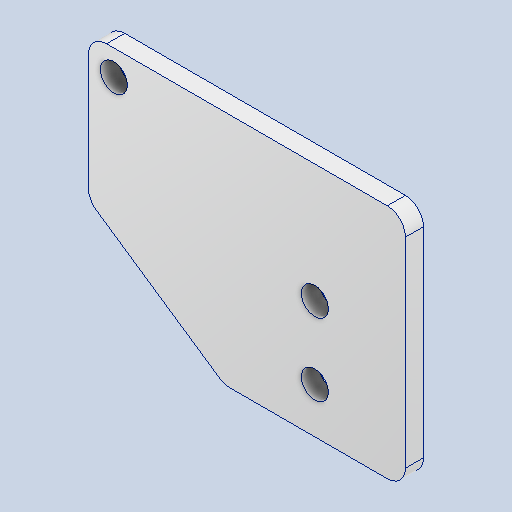
# Autodesk Inventor part: dribl-v1-Plate-12
Saved by Autodesk Inventor 2025.2 (Build 292293000, 293)
## iProperties
Created: 2025-01-15
Part Number: dribl-v1-Plate-12
Material: アルミニウム 6061
Document SubType Name: Modeling
Designer: haruy
Density: 2.7 g/cm^3
Appearance: アルミニウム - フラット
Author: haruy
Autodesk Inventor part; units mm, degrees
ref_plane "YZ Plane" through (0, 0, 0) normal (1, 0, 0) x (0, 1, 0)
ref_plane "XZ Plane" through (0, 0, 0) normal (0, 1, 0) x (-1, 0, 0)
ref_plane "XY Plane" through (0, 0, 0) normal (0, 0, 1) x (1, 0, 0)
sketch "スケッチ1" plane through (0, 0, 0) normal (0, 0, 1) x (1, 0, 0)
  line L0 (207.1172, 661.0147) -> (207.1172, -646.9853)
  line L1 (207.1172, 628.8147) -> (187.1172, 628.8147)
  line L2 (187.1172, 661.0147) -> (187.1172, -646.9853)
  line L3 (187.1172, 25.0147) -> (207.1172, 25.0147)
  line L4 (187.1172, -646.9853) -> (207.1172, -646.9853)
  line L5 (187.1172, 661.0147) -> (207.1172, 661.0147)
  line L6 (172.1172, 612.9147) -> (199.9172, 612.9147)
  line L7 (199.9172, 612.9147) -> (199.9172, 628.8147)
  line L8 (199.9172, 628.8147) -> (172.1172, 628.8147)
  line L9 (172.1172, 628.8147) -> (172.1172, 612.9147)
  circle A0 centre (174.9172, 615.7147) radius 1.5
  circle A1 centre (197.1172, 626.0147) radius 1.5
  circle A2 centre (197.1172, 634.0147) radius 1.5
  line L10 (172.1172, 79.1147) -> (199.9172, 79.1147)
  line L11 (199.9172, 79.1147) -> (199.9172, 63.2147)
  line L12 (199.9172, 63.2147) -> (172.1172, 63.2147)
  line L13 (172.1172, 63.2147) -> (172.1172, 79.1147)
  circle A3 centre (174.9172, 76.3147) radius 1.5
  circle A4 centre (197.1172, 66.0147) radius 1.5
  circle A5 centre (197.1172, 58.0147) radius 1.5
  line L14 (187.1172, 639.0147) -> (207.1172, 639.0147)
  line L15 (199.9172, 612.9147) -> (207.1172, 612.9147)
  line L16 (207.1172, 612.9147) -> (207.1172, 639.0147)
  line L17 (187.1172, 639.0147) -> (172.1172, 628.8147)
  line L18 (187.1172, 53.0147) -> (207.1172, 53.0147)
  line L19 (199.9172, 79.1147) -> (207.1172, 79.1147)
  line L20 (207.1172, 79.1147) -> (207.1172, 53.0147)
  line L21 (187.1172, 53.0147) -> (172.1172, 63.2147)
  point P0 (0, 0)
  point P1 (-212.8828, -214.6519)
  dimension "d0" = 672
  dimension "d1" = 27.8
  dimension "d2" = 15.9
  dimension "d3" = 3
  dimension "d4" = 3
  dimension "d5" = 2.8
  dimension "d6" = 2.8
  dimension "d7" = 2.8
  dimension "d8" = 2.8
  dimension "d9" = 0
  dimension "d10" = 10
  dimension "d11" = 3
  dimension "d12" = 8
  dimension "d13" = 10
  dimension "d14" = 27
  dimension "d15" = 27.8
  dimension "d16" = 15.9
  dimension "d17" = 3
  dimension "d18" = 3
  dimension "d19" = 2.8
  dimension "d20" = 2.8
  dimension "d21" = 2.8
  dimension "d22" = 2.8
  dimension "d23" = 10
  dimension "d24" = 560
  dimension "d25" = 3
  dimension "d26" = 8
  dimension "d27" = 10
  dimension "d28" = 5
  dimension "d29" = 5
  constraints: 44 end point, 10 point on line, 7 perpendicular, 6 centre point, 5 horizontal, 4 parallel
  measures "d0" distance between parallel lines of L4 L3
  measures "d1" distance of L8.end L7.end
  measures "d2" distance of L7.end L6.end
  measures "d3" diameter of A0
  measures "d4" diameter of A1
  measures "d5" distance from line of A0.centre L6
  measures "d6" distance from line of A0.centre L9
  measures "d7" distance from line of A1.centre L8
  measures "d8" distance from line of L7 A1.centre
  measures "d9" distance between parallel lines of L1 L8
  measures "d10" distance from line of A1.centre L2
  measures "d11" diameter of A2
  measures "d12" distance of A1.centre A2.centre
  measures "d13" distance from line of L2 A2.centre
  measures "d14" distance from line of A2.centre L5
  measures "d15" distance of L11.end L12.end
  measures "d16" distance of L10.end L11.end
  measures "d17" diameter of A3
  measures "d18" diameter of A4
  measures "d19" distance from line of A3.centre L10
  measures "d20" distance from line of A3.centre L13
  measures "d21" distance from line of A4.centre L12
  measures "d22" distance from line of L11 A4.centre
  measures "d23" distance from line of L0 A4.centre
  measures "d24" distance of A1.centre A4.centre
  measures "d25" diameter of A5
  measures "d26" distance of A5.centre A4.centre
  measures "d27" distance from line of A5.centre L2
  measures "d28" distance from line of A2.centre L14
  measures "d29" distance from line of A5.centre L18
extrude "押し出し1" add sketch "スケッチ1" against normal blind 2 contours L0 L18 L2 L12 L11 L19 | L11 L12 L2 L10 | L2 L12 L13 L10 | L21 L12 L2
fillet "フィレット1" radius 2 5 edges at (172.1172, 79.1147, -1) (172.1172, 63.2147, -1) (187.1172, 53.0147, -1) (207.1172, 53.0147, -1) (207.1172, 79.1147, -1)
equation "\"d6\" = d5"
equation "\"d7\" = d5"
equation "\"d8\" = d5"
equation "\"d20\" = d19"
equation "\"d21\" = d19"
equation "\"d22\" = d19"
